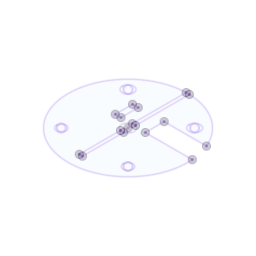
3-layer hub v2 (Autodesk Fusion 360 design; units mm, degrees)
Autodesk Fusion 360 part; units mm, degrees
sketch "layout" plane through (0, 0, 0) normal (0, 1, 0) x (1, 0, 0)
  circle A0 centre (0, 0) radius 1.95
  line L0 (-5.1815, 4.5) -> (5.2405, 4.5) construction
  line L1 (0.5, -14.9917) -> (0.5, 19.1614)
  line L2 (-0.5, -14.9917) -> (-0.5, 19.2062)
  line L3 (-4, 1.75) -> (-5.8, 1.75)
  line L4 (-5.8, 1.75) -> (-5.8, 7.25)
  line L5 (-5.8, 7.25) -> (-4, 7.25)
  line L6 (-4, 7.25) -> (-4, 1.75)
  line L7 (-4, 1.75) -> (-5.8, 7.25) construction
  line L8 (-5.8, 1.75) -> (-4, 7.25) construction
  line L9 (24, 1.5) -> (4, 1.5)
  line L10 (4, 1.5) -> (4, 7.5)
  line L11 (4, 7.5) -> (24, 7.5)
  line L12 (24, 7.5) -> (24, 1.5)
  line L13 (24, 1.5) -> (4, 7.5) construction
  line L14 (4, 1.5) -> (24, 7.5) construction
  line L15 (25.0295, 3) -> (-24.9705, 3)
  line L16 (-24.9705, 3) -> (-24.9705, 6)
  line L17 (-24.9705, 6) -> (25.0295, 6)
  line L18 (25.0295, 6) -> (25.0295, 3)
  line L19 (25.0295, 3) -> (-24.9705, 6) construction
  line L20 (-24.9705, 3) -> (25.0295, 6) construction
  line L21 (-7.8, 7.25) -> (-7.8, 1.75)
  line L22 (0.5, -14.9917) -> (33.9874, -14.9917) construction
  line L23 (0, 0) -> (35.3553, -35.3553) construction
  line L24 (0, 0) -> (50, 0) construction
  line L25 (0, 0) -> (35.3553, 35.3553) construction
  line L26 (0, 0) -> (-35.3553, 35.3553) construction
  line L27 (0, 0) -> (-35.3553, -35.3553) construction
  circle A1 centre (10.6066, 10.6066) radius 1.8
  circle A2 centre (10.6066, 10.6066) radius 3 construction
  circle A3 centre (0, 0) radius 15 construction
  circle A4 centre (-10.6066, 10.6066) radius 1.8
  circle A5 centre (10.6066, -10.6066) radius 1.5
  circle A6 centre (-10.6066, -10.6066) radius 1.5
  circle A7 centre (0, 0) radius 19
  line L28 (4, 7.5) -> (-4, 7.5)
  line L29 (-4, 7.5) -> (-4, 7.25)
  line L30 (-0.5, -14.9917) -> (0.5, -14.9917)
  point P0 (-4.9, 4.5)
  point P1 (14, 4.5)
  point P2 (0.0295, 4.5)
  dimension "d6" = 3.9
  dimension "d7" = 4.5
  dimension "d9" = 0.5
  dimension "d10" = 0.5
  dimension "d13" = 1.8
  dimension "d14" = 5.5
  dimension "d15" = 20
  dimension "d16" = 6
  dimension "d17" = 4
  dimension "d18" = 4
  dimension "d19" = 50
  dimension "d20" = 3
  dimension "d22" = 2
  dimension "d24" = 45
  dimension "d25" = 50
  dimension "d27" = 360
  dimension "d28" = 3.6
  dimension "d29" = 15
  dimension "d30" = 6
  dimension "d32" = 3.6
  dimension "d33" = 3
  dimension "d34" = 3
  dimension "d35" = 38
  constraint coincident A0.centre L23.start
  constraint horizontal L0
  constraint perpendicular L0 L1
  constraint parallel L1 L2
  constraint horizontal L3
  constraint perpendicular L3 L4
  constraint parallel L3 L5
  constraint parallel L4 L6
  constraint coincident L7 P0
  constraint coincident L8 P0
  constraint coincident L0 P0
  constraint horizontal L9
  constraint perpendicular L9 L10
  constraint parallel L9 L11
  constraint parallel L10 L12
  constraint coincident L13 P1
  constraint coincident L14 P1
  constraint coincident L0 P1
  constraint horizontal L15
  constraint perpendicular L15 L16
  constraint parallel L15 L17
  constraint parallel L16 L18
  constraint coincident L19 P2
  constraint coincident L20 P2
  constraint midpoint L0 P2
  constraint perpendicular L15 L21
  constraint horizontal L22
  constraint horizontal L24
  constraint coincident L25 A1.centre
  constraint concentric A1 A2
  constraint concentric A0 A3
  constraint coincident A1.centre A3
  constraint coincident A3 A4.centre
  constraint coincident L26 A4.centre
  constraint coincident A3 A5.centre
  constraint coincident L23 A5.centre
  constraint coincident A3 A6.centre
  constraint coincident L27 A6.centre
  constraint perpendicular L6 L28
  constraint perpendicular L5 L29
  constraint coincident L1.start A3
  constraint coincident L2.start A3
  measures "d6" diameter of A0
  measures "d7" distance of A0.centre L0
  measures "d9" distance of A0.centre L1
  measures "d10" distance of A0.centre L2
  measures "d13" distance of L4.end L5.end
  measures "d14" distance of L3.end L4.end
  measures "d15" distance of L10.end L11.end
  measures "d16" distance of L9.end L10.end
  measures "d17" distance of A0.centre L6
  measures "d18" distance of A0.centre L10
  measures "d19" distance of L16.end L17.end
  measures "d20" distance of L15.end L16.end
  measures "d22" distance of L4 L21
  measures "d24" angle of L23 L24
  measures "d25" distance of A0.centre L23.end
  measures "d28" diameter of A1
  measures "d29" distance of A0.centre A1.centre
  measures "d30" diameter of A2
  measures "d32" diameter of A4
  measures "d33" diameter of A5
  measures "d34" diameter of A6
  measures "d35" diameter of A7
extrude "Extrude3" add sketch "layout" along normal blind 3 from surface at 1.5 contours A0 L1 L2 L3 L4 L6 L9 L10 L15 A7 L30 | L1 L10 L15 L17 | L2 L6 L15 L17 | L1 L10 L17 L28 | L2 L6 L17 L28 L29 | L1 L11 A7 L28 | L2 L4 L5 L17 A7 L28 L29 | L4 L15 L17 L21 | L15 L17 L21 A7 makes body 1
extrude "Extrude1" add sketch "layout" along normal mid plane 3 separate body contours A0 L1 L2 L3 L4 L6 L9 L10 L15 A7 L30 makes body 2
extrude "Extrude2" add sketch "layout" along normal mid plane 3 separate body contours L1 L2 A7 L28 | L1 L11 A7 L28 | L2 L4 L5 L17 A7 L28 L29 makes body 3
sketch "clean outer plate" plane through (0, 0, 0) normal (0, 1, 0) x (-1, 0, 0)
  circle A0 centre (-10.6066, 10.6066) radius 1.5
  circle A1 centre (10.6066, 10.6066) radius 1.5
  line L0 (5.8, -7.25) -> (4, -7.25)
  line L1 (4, -7.25) -> (4, -1.75)
  line L2 (4, -1.75) -> (5.8, -1.75)
  line L3 (5.8, -1.75) -> (5.8, -7.25)
  circle A2 centre (-10.6066, -10.6066) radius 1.8
  circle A3 centre (10.6066, -10.6066) radius 1.8
  line L4 (0.5, -1.8848) -> (0.5, -18.9934)
  arc A4 (0.5, -18.9934) -> (-18.9407, -1.5) centre (0, 0) ccw
  line L5 (-18.9407, -1.5) -> (-4, -1.5)
  line L6 (-4, -1.5) -> (-4, -7.5)
  line L7 (-4, -7.5) -> (-17.4571, -7.5)
  arc A5 (-17.4571, -7.5) -> (-0.5, -18.9934) centre (0, 0) ccw
  line L8 (-0.5, -18.9934) -> (-0.5, -1.8848)
  arc A6 (-0.5, 1.8848) -> (-0.5, -1.8848) centre (0, 0) ccw
  line L9 (-0.5, 1.8848) -> (-0.5, 14.9917)
  line L10 (-0.5, 14.9917) -> (0.5, 14.9917)
  line L11 (0.5, 14.9917) -> (0.5, 1.8848)
  arc A7 (0.5, -1.8848) -> (0.5, 1.8848) centre (0, 0) ccw
sketch "clean inner bottom" plane through (0, 1.5, 0) normal (0, 1, 0) x (-1, 0, 0)
  circle A0 centre (-10.6066, 10.6066) radius 1.5
  circle A1 centre (10.6066, 10.6066) radius 1.5
  line L0 (0.5, -1.8848) -> (0.5, -3)
  line L1 (0.5, -3) -> (4, -3)
  line L2 (4, -3) -> (4, -1.75)
  line L3 (4, -1.75) -> (5.8, -1.75)
  line L4 (5.8, -1.75) -> (5.8, -3)
  line L5 (5.8, -3) -> (18.7617, -3)
  arc A2 (18.7617, -3) -> (-18.9407, -1.5) centre (0, 0) ccw
  line L6 (-18.9407, -1.5) -> (-4, -1.5)
  line L7 (-4, -1.5) -> (-4, -3)
  line L8 (-4, -3) -> (-0.5, -3)
  line L9 (-0.5, -3) -> (-0.5, -1.8848)
  arc A3 (-0.5, 1.8848) -> (-0.5, -1.8848) centre (0, 0) ccw
  line L10 (-0.5, 1.8848) -> (-0.5, 14.9917)
  line L11 (-0.5, 14.9917) -> (0.5, 14.9917)
  line L12 (0.5, 14.9917) -> (0.5, 1.8848)
  arc A4 (0.5, -1.8848) -> (0.5, 1.8848) centre (0, 0) ccw
sketch "clean inner top" plane through (0, 1.5, 0) normal (0, 1, 0) x (-1, 0, 0)
  circle A0 centre (10.6066, -10.6066) radius 1.8
  circle A1 centre (-10.6066, -10.6066) radius 1.8
  line L0 (4, -7.5) -> (-17.4571, -7.5)
  arc A2 (-17.4571, -7.5) -> (18.0278, -6) centre (0, 0) ccw
  line L1 (18.0278, -6) -> (5.8, -6)
  line L2 (5.8, -6) -> (5.8, -7.25)
  line L3 (5.8, -7.25) -> (4, -7.25)
  line L4 (4, -7.25) -> (4, -7.5)
hidden bodies 1 2 3
equation "shaftDia = 4 mm"
equation "kerfOffset = 0.1 mm"
equation "boltDia = 3 mm"
equation "nutSide = 5.5 mm"
equation "washerHeight = 6 mm"
equation "d6 = shaftDia - kerfOffset"
equation "d7 = 1 mm + shaftDia / 2 + boltDia / 2"
equation "slotWidth = 1 mm"
equation "d9 = slotWidth / 2"
equation "d10 = slotWidth / 2"
equation "nutThickness = 1.8 mm"
equation "clampFaceFromCenter = 4 mm"
equation "d13 = nutThickness"
equation "d14 = nutSide"
equation "d16 = washerHeight"
equation "d17 = clampFaceFromCenter"
equation "d18 = clampFaceFromCenter"
equation "d20 = boltDia"
equation "d28 = boltDia + boltExtraClearance"
equation "d30 = washerHeight"
equation "boltExtraClearance = 0.6 mm"
equation "d32 = boltDia + boltExtraClearance"
equation "d33 = boltDia"
equation "d34 = boltDia"
equation "d36 = boltDia / 2"
equation "d38 = boltDia / 2"
equation "d40 = boltDia / 2"
equation "d41 = boltDia"
named bodies: "inner bottom", "inner top", "outer plate"
